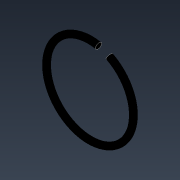
# Autodesk Inventor part: Pierścień ustalający
Saved by Autodesk Inventor 2022 (Build 260153000, 153)
## iProperties
Created: 2023-05-20
Part Number: Pierścień ustalający
Material: Generic
Document SubType Name: Modeling
Designer: wikto
Density: 1 g/cm^3
Appearance: Anodized - Black
Author: wikto
Autodesk Inventor part; units mm, degrees
ref_plane "YZ Plane" through (0, 0, 0) normal (1, 0, 0) x (0, 1, 0)
ref_plane "XZ Plane" through (0, 0, 0) normal (0, 1, 0) x (-1, 0, 0)
sketch "Sketch1" plane through (0, 0, 0) normal (0, 0, 1) x (1, 0, 0)
  arc A0 (4.1742, 20.581) -> (9.3587, 18.7993) centre (0, 0) ccw
  line L0 (4.1742, 20.581) -> (0, 0) construction
  line L1 (0, 0) -> (9.3587, 18.7993) construction
  dimension "d0" = 15
  dimension "d1" = 42
  constraints: 4 end point, 2 point on circle, 1 centre point, 1 coincident
  measures "d0" angle of L1 L0
  measures "d1" diameter of A0
ref_plane "Work Plane1" through (4.1742, 20.581, 0) normal (-0.98, 0.1988, 0) x (-0.1988, -0.98, 0)
sketch "Sketch2" plane through (4.1742, 20.581, 0) normal (-0.98, 0.1988, 0) x (-0.1988, -0.98, 0)
  circle A0 centre (0, 0) radius 1.5
  point P0 (21, 0)
  dimension "d2" = 3
  constraints: 1 centre point
  measures "d2" diameter of A0
sweep "Sweep1" add profiles "Sketch2" path "Sketch1"
body "Solid1"
